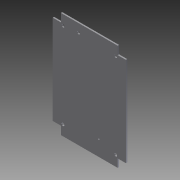
# Autodesk Inventor part: power supply pcb
Saved by Autodesk Inventor 2012 (Build 160160000, 160)
## iProperties
Created: 2017-06-15
Part Number: power supply pcb
Material: Default
Document SubType Name: Modeling
Designer: Brandon
Density: 1 g/cm^3
Author: Brandon
Autodesk Inventor part; units mm, degrees
ref_plane "YZ Plane" through (0, 0, 0) normal (1, 0, 0) x (0, 1, 0)
ref_plane "XZ Plane" through (0, 0, 0) normal (0, 1, 0) x (-1, 0, 0)
ref_plane "XY Plane" through (0, 0, 0) normal (0, 0, 1) x (1, 0, 0)
sketch "Sketch1" plane through (0, 0, 0) normal (0, 0, 1) x (1, 0, 0)
  line L0 (-33.02, 52.07) -> (33.02, 52.07)
  line L1 (33.02, 52.07) -> (33.02, -52.07)
  line L2 (33.02, -52.07) -> (-33.02, -52.07)
  line L3 (-33.02, -52.07) -> (-33.02, 52.07)
  line L4 (-42.545, 61.595) -> (42.545, 61.595)
  line L5 (42.545, 61.595) -> (42.545, -61.595)
  line L6 (42.545, -61.595) -> (-42.545, -61.595)
  line L7 (-42.545, -61.595) -> (-42.545, 61.595)
  line L8 (-33.02, 52.07) -> (33.02, 52.07)
  line L9 (33.02, 52.07) -> (33.02, 61.595)
  line L10 (33.02, 61.595) -> (-33.02, 61.595)
  line L11 (-33.02, 61.595) -> (-33.02, 52.07)
  line L12 (-33.02, 52.07) -> (-42.545, 52.07)
  line L13 (-42.545, 52.07) -> (-42.545, -52.07)
  line L14 (-42.545, -52.07) -> (-33.02, -52.07)
  line L15 (-33.02, -52.07) -> (-33.02, 52.07)
  line L16 (33.02, -52.07) -> (42.545, -52.07)
  line L17 (42.545, -52.07) -> (42.545, 52.07)
  line L18 (42.545, 52.07) -> (33.02, 52.07)
  line L19 (33.02, 52.07) -> (33.02, -52.07)
  line L20 (-33.02, -52.07) -> (33.02, -52.07)
  line L21 (33.02, -52.07) -> (33.02, -61.595)
  line L22 (33.02, -61.595) -> (-33.02, -61.595)
  line L23 (-33.02, -61.595) -> (-33.02, -52.07)
  point P0 (0, 0)
  dimension "d0" = 104.14
  dimension "d1" = 123.19
  dimension "d2" = 66.04
  dimension "d3" = 85.09
  dimension "d4" = 52.07
  dimension "d5" = 33.02
  dimension "d6" = 61.595
  dimension "d7" = 42.545
  constraints: 48 end point, 12 parallel, 6 horizontal, 6 perpendicular, 4 point on line
  measures "d0" distance of L2.end L0.start
  measures "d1" distance of L6.end L4.start
  measures "d2" distance of L0.start L0.end
  measures "d3" distance of L4.start L4.end
  measures "d4" distance from line of L0 point (0, 0)
  measures "d5" distance from line of L3 point (0, 0)
  measures "d6" distance from line of point (0, 0) L4
  measures "d7" distance from line of L7 point (0, 0)
extrude "Extrusion1" add sketch "Sketch1" along normal blind 1.5748 contours L11 L4 L9 L0 | L0 L1 L2 L3 | L3 L14 L7 L12 | L18 L5 L16 L1 | L2 L21 L6 L23
hole "Hole1" at (30.6324, 49.6824, 1.5748) direction (0, 0, -1) diameter 3.175 end through all
hole "Hole2" at (-30.6578, 49.7078, 1.5748) direction (0, 0, -1) diameter 3.175 end through all
hole "Hole3" at (-30.6578, -49.7078, 1.5748) direction (0, 0, -1) diameter 3.175 end through all
hole "Hole4" at (30.6578, -49.7078, 1.5748) direction (0, 0, -1) diameter 3.175 end through all
hole "Hole5" at (10.8712, -43.4848, 1.5748) direction (0, 0, -1) diameter 2.0066 end through all
hole "Hole6" at (-12.4968, 51.8414, 1.5748) direction (0, 0, -1) diameter 3.175 end through all
equation "\"d4\" = 0.5 * d0"
equation "\"d5\" = 0.5 * d2"
equation "\"d6\" = 0.5 * d1"
equation "\"d7\" = 0.5 * d3"
body "Solid1"
